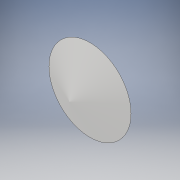
# Autodesk Inventor part: Rotation
Saved by Autodesk Inventor 2018 (Build 220112000, 112)
## iProperties
Created: 2017-07-02
Part Number: Rotation
Material: Generisch
Document SubType Name: Modeling
Designer: Ich
Density: 1 g/cm^3
Appearance: Vorgabe
Author: Ich
Autodesk Inventor part; units mm, degrees
ref_plane "YZ Plane" through (0, 0, 0) normal (1, 0, 0) x (0, 1, 0)
ref_plane "XZ Plane" through (0, 0, 0) normal (0, 1, 0) x (-1, 0, 0)
ref_plane "XY Plane" through (0, 0, 0) normal (0, 0, 1) x (1, 0, 0)
sketch "Skizze1" plane through (0, 0, 0) normal (0, 0, 1) x (1, 0, 0)
  line L0 (0, 20) -> (0, -20)
  line L1 (0, -20) -> (40, 0)
  line L2 (40, 0) -> (0, 20)
  line L3 (40, 0) -> (8.4479, 0) construction
  line L4 (-8, 0) -> (48, 0) construction
  line L5 (0, -28) -> (0, 28) construction
  point P0 (0, 0)
  dimension "d4" = 40
  dimension "d5" = 40
  constraints: 8 end point, 2 collinear, 1 horizontal, 1 symmetric about line, 1 vertical
  measures "d4" distance from line of L0 L1.end
  measures "d5" distance of L0.start L0.end
revolve "Umdrehung1" add sketch "Skizze1" angle 360 about axis through (0, 20, 0) along (0, -1, 0)
equation "\"d5\" = d4"
